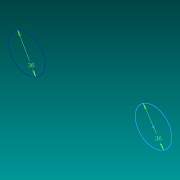
# Autodesk Inventor part: 皮带4
Saved by Autodesk Inventor 2021 (Build 250183000, 183)
## iProperties
Created: 2025-04-17
Part Number: 皮带4
Material: 常规
Document SubType Name: Modeling
Designer: 86155
Density: 1 g/cm^3
Appearance: 默认
Author: 86155
Autodesk Inventor part; units mm, degrees
ref_plane "YZ Plane" through (0, 0, 0) normal (1, 0, 0) x (0, 1, 0)
ref_plane "XZ Plane" through (0, 0, 0) normal (0, 1, 0) x (-1, 0, 0)
ref_plane "XY Plane" through (0, 0, 0) normal (0, 0, 1) x (1, 0, 0)
sketch "草图1" plane through (0, 0, 0) normal (0, 0, 1) x (1, 0, 0)
  arc A0 (0, 18) -> (0, -18) centre (0, 0) ccw
  arc A1 (720, -18) -> (720, 18) centre (720, 0) ccw
  line L0 (0, 18) -> (720, 18)
  line L1 (720, -18) -> (0, -18)
  line L2 (720, 20) -> (0, 20)
  arc A2 (0, 20) -> (0, -20) centre (0, 0) ccw
  line L3 (0, -20) -> (720, -20)
  arc A3 (720, -20) -> (720, 20) centre (720, 0) ccw
  dimension "d0" = 36
  dimension "d1" = 36
  dimension "d2" = 720
  dimension "d3" = 2
  constraints: 8 end point, 8 point on circle, 4 centre point, 3 tangent, 1 coincident, 3 other
  measures "d0" diameter of A0
  measures "d1" diameter of A1
  measures "d2" distance of A1.centre A0.centre
  measures "d3" distance between parallel lines of L0 L2
extrude "拉伸1" add sketch "草图1" along normal blind 10
